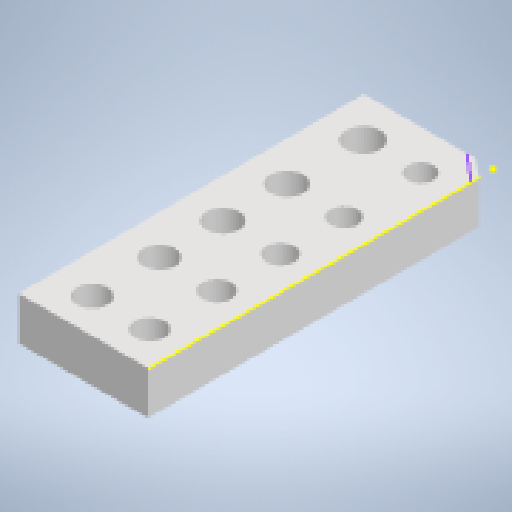
# Autodesk Inventor part: m3_sizing_tests
Saved by Autodesk Inventor 2023 (Build 270158000, 158)
## iProperties
Created: 2022-10-04
Part Number: m3_sizing_tests
Material: Generic
Document SubType Name: Modeling
Designer: carso
Density: 1 g/cm^3
Appearance: Default
Author: carso
Autodesk Inventor part; units mm, degrees
ref_plane "YZ Plane" through (0, 0, 0) normal (1, 0, 0) x (0, 1, 0)
ref_plane "XZ Plane" through (0, 0, 0) normal (0, 1, 0) x (-1, 0, 0)
ref_plane "XY Plane" through (0, 0, 0) normal (0, 0, 1) x (1, 0, 0)
sketch "Sketch1" plane through (0, 0, 0) normal (0, 1, 0) x (-1, 0, 0)
  line L0 (0, 0) -> (15, 0)
  line L1 (15, 0) -> (15, 40)
  line L2 (15, 40) -> (0, 40)
  line L3 (0, 40) -> (0, 0)
  circle A0 centre (3.7979, 4.6387) radius 1.5
  circle A1 centre (3.7979, 13.4768) radius 1.55
  circle A2 centre (3.7979, 20.9025) radius 1.6
  circle A3 centre (3.7979, 28.2372) radius 1.65
  circle A4 centre (3.7979, 36.0274) radius 1.7
  circle A5 centre (10.4492, 36.0274) radius 1.75
  circle A6 centre (10.4492, 28.2372) radius 1.8
  circle A7 centre (10.4492, 20.9025) radius 1.85
  circle A8 centre (10.4492, 13.4768) radius 1.9
  circle A9 centre (10.4492, 4.6387) radius 1.95
  line L4 (2.0979, 0) -> (0, 1.698)
  point P0 (7.5, 40)
  dimension "d0" = 3
  dimension "d1" = 3.1
  dimension "d2" = 3.2
  dimension "d3" = 3.3
  dimension "d4" = 3.4
  dimension "d5" = 3.5
  dimension "d6" = 3.6
  dimension "d7" = 3.7
  dimension "d8" = 3.8
  dimension "d9" = 3.9
  dimension "d10" = 40
  dimension "d11" = 15
  constraints: 10 centre point, 10 end point, 2 parallel, 2 point on line, 1 horizontal, 1 midpoint, 1 perpendicular
  measures "d0" diameter of A0
  measures "d1" diameter of A1
  measures "d2" diameter of A2
  measures "d3" diameter of A3
  measures "d4" diameter of A4
  measures "d5" diameter of A5
  measures "d6" diameter of A6
  measures "d7" diameter of A7
  measures "d8" diameter of A8
  measures "d9" diameter of A9
  measures "d10" distance from line of L0 point (7.5, 40)
  measures "d11" distance of L1.end L2.end
extrude "Extrusion1" add sketch "Sketch1" along normal blind 5 contours L4 L3 L2 L1 L0
sketch "Sketch2" plane through (0, 5, 0) normal (0, 1, 0) x (1, 0, 0)
  line L0 (0, -40) -> (0, -1.698) projected
  line L1 (0, -1.698) -> (-2.0979, 0) projected
  line L2 (-2.0979, 0) -> (0, -1.698)
  line L3 (0, -1.698) -> (0, -2.698)
  line L4 (-2.0979, 0) -> (-3.0979, 0)
  line L5 (-2.0979, 0) -> (-15, 0) projected
  line L6 (-3.0979, 0) -> (0, -2.698)
  point P0 (0, 0)
  dimension "d14" = 1
  dimension "d15" = 1
  constraints: 8 end point, 2 point on line, 1 collinear
  measures "d14" distance of L0.end L3.end
  measures "d15" distance of L1.end L4.end
extrude "Extrusion2" cut sketch "Sketch2" against normal blind 2.5
body "Solid1"
